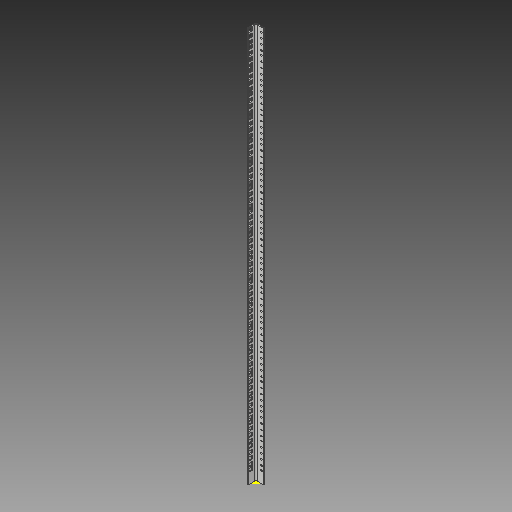
# Autodesk Inventor part: squareHoleRail20U
Saved by Autodesk Inventor 2017 (Build 210142000, 142)
## iProperties
Created: 2016-08-02
Part Number: squareHoleRail20U
Material: Generic
Document SubType Name: Sheet Metal
Designer: Zuhra Abdurashidova
Density: 1 g/cm^3
Sheet Metal Rule: Default
Appearance: Default
Author: Zuhra Abdurashidova
Autodesk Inventor part; units mm, degrees
note: some values were not read from the file. Chosen so that the rebuilt part matches the saved one: flange form of "Plate1".
ref_plane "YZ Plane" through (0, 0, 0) normal (1, 0, 0) x (0, 1, 0)
ref_plane "XZ Plane" through (0, 0, 0) normal (0, 1, 0) x (-1, 0, 0)
ref_plane "XY Plane" through (0, 0, 0) normal (0, 0, 1) x (1, 0, 0)
sketch "Sketch1" plane through (0, 0, 0) normal (0, 1, 0) x (-1, 0, 0)
  line L0 (0, 25.4) -> (0, 0)
  line L1 (0, 0) -> (-25.4, 0)
  dimension "d0" = 25.4
  dimension "d1" = 25.4
  measures "d0" distance of L0.start L0.end
  measures "d1" distance of L0.end L1.end
contour flange "Contour Flange1" sketch "Sketch1" thickness 3.048 bend radius 3.048 width 1174.75 along (0, 1, 0) mid plane no both sides no wall seen from (0, 0, 12.7) lies toward (1, 0, 0) curves L0 L1
bend "Bend1"
corner "Corner1"
sketch "Sketch2" plane through (0, 0, 25.4) normal (-1, 0, 0) x (0, 0, 1)
  line L0 (0, 1174.75) -> (0, 0) projected
  line L1 (-11.35, 1163.4) -> (-1.35, 1163.4)
  line L2 (-1.35, 1163.4) -> (-1.35, 1173.4)
  line L3 (-1.35, 1173.4) -> (-11.35, 1173.4)
  line L4 (-11.35, 1173.4) -> (-11.35, 1163.4)
  line L5 (-11.35, 1163.4) -> (-1.35, 1173.4) construction
  line L6 (-1.35, 1163.4) -> (-11.35, 1173.4) construction
  line L7 (-19.304, 1174.75) -> (0, 1174.75) projected
  line L8 (-11.35, 1147.5) -> (-1.35, 1147.5)
  line L9 (-1.35, 1147.5) -> (-1.35, 1157.5)
  line L10 (-1.35, 1157.5) -> (-11.35, 1157.5)
  line L11 (-11.35, 1157.5) -> (-11.35, 1147.5)
  line L12 (-11.35, 1147.5) -> (-1.35, 1157.5) construction
  line L13 (-1.35, 1147.5) -> (-11.35, 1157.5) construction
  line L14 (-11.35, 1131.6) -> (-1.35, 1131.6)
  line L15 (-1.35, 1131.6) -> (-1.35, 1141.6)
  line L16 (-1.35, 1141.6) -> (-11.35, 1141.6)
  line L17 (-11.35, 1141.6) -> (-11.35, 1131.6)
  line L18 (-11.35, 1131.6) -> (-1.35, 1141.6) construction
  line L19 (-1.35, 1131.6) -> (-11.35, 1141.6) construction
  line L20 (-11.35, 1118.9) -> (-1.35, 1118.9)
  line L21 (-1.35, 1118.9) -> (-1.35, 1128.9)
  line L22 (-1.35, 1128.9) -> (-11.35, 1128.9)
  line L23 (-11.35, 1128.9) -> (-11.35, 1118.9)
  line L24 (-11.35, 1118.9) -> (-1.35, 1128.9) construction
  line L25 (-1.35, 1118.9) -> (-11.35, 1128.9) construction
  point P0 (-25.4, 0)
  point P1 (-6.35, 1168.4)
  point P2 (-6.35, 1152.5)
  point P3 (-6.35, 1136.6)
  point P4 (-6.35, 1123.9)
  dimension "d13" = 6.35
  dimension "d14" = 6.35
  dimension "d15" = 10
  dimension "d16" = 10
  dimension "d17" = 15.9
  dimension "d18" = 10
  dimension "d19" = 10
  dimension "d20" = 15.9
  dimension "d21" = 10
  dimension "d22" = 10
  dimension "d23" = 12.7
  dimension "d24" = 10
  dimension "d25" = 10
  constraints: 48 end point, 8 midpoint, 8 parallel, 4 horizontal, 4 perpendicular
  measures "d13" distance from line of L0 point (-6.35, 1168.4)
  measures "d14" distance from line of L7 point (-6.35, 1168.4)
  measures "d15" distance of L3.end L1.start
  measures "d16" distance of L2.end L3.end
  measures "d17" distance of point (-6.35, 1152.5) point (-6.35, 1168.4)
  measures "d18" distance of L9.end L10.end
  measures "d19" distance of L8.end L9.end
  measures "d20" distance of point (-6.35, 1152.5) point (-6.35, 1136.6)
  measures "d21" distance of L15.end L16.end
  measures "d22" distance of L14.end L15.end
  measures "d23" distance of point (-6.35, 1123.9) point (-6.35, 1136.6)
  measures "d24" distance of L20.end L21.end
  measures "d25" distance of L21.end L22.end
extrude "Extrusion1" cut sketch "Sketch2" against normal blind 6
pattern_linear "Rectangular Pattern1" count 19 spacing 60.4 along (0, -1, 0) of "Extrusion1"
sketch "Sketch3" plane through (25.4, 0, 0) normal (0, 0, -1) x (-1, 0, 0)
  point P0 (25.4, 0)
sketch "Sketch4" plane through (25.4, 0, 0) normal (0, 0, -1) x (-1, 0, 0)
  point P0 (25.4, 0)
sketch "10-32 holes" plane through (25.4, 0, 0) normal (0, 0, -1) x (-1, 0, 0)
  circle A0 centre (6.35, 1162.05) radius 2.415
  line L0 (0, 1174.75) -> (19.304, 1174.75) projected
  line L1 (0, 0) -> (0, 1174.75) projected
  circle A1 centre (6.35, 1146.15) radius 2.415
  circle A2 centre (6.35, 1130.25) radius 2.415
  circle A3 centre (6.35, 1114.35) radius 2.415
  circle A4 centre (6.35, 1101.65) radius 2.415
  point P0 (25.4, 0)
  dimension "d31" = 4.83
  dimension "d32" = 12.7
  dimension "d33" = 6.35
  dimension "d34" = 4.83
  dimension "d35" = 15.9
  dimension "d36" = 6.35
  dimension "d37" = 4.83
  dimension "d38" = 15.9
  dimension "d39" = 4.83
  dimension "d40" = 15.9
  dimension "d41" = 4.83
  dimension "d42" = 12.7
  constraints: 5 centre point, 4 coincident
  measures "d31" diameter of A0
  measures "d32" distance from line of L0 A0.centre
  measures "d33" distance from line of L1 A0.centre
  measures "d34" diameter of A1
  measures "d35" distance of A0.centre A1.centre
  measures "d36" distance from line of L1 A1.centre
  measures "d37" diameter of A2
  measures "d38" distance of A1.centre A2.centre
  measures "d39" diameter of A3
  measures "d40" distance of A2.centre point (6.35, 1114.35)
  measures "d41" diameter of A4
  measures "d42" distance of A3.centre A4.centre
extrude "Extrusion2" cut sketch "10-32 holes" against normal blind 10
pattern_linear "Rectangular Pattern2" count 15 spacing 76.3 along (0, -1, 0) of "Extrusion2"
equation "\"d3\" = BendReliefWidth"
equation "\"d4\" = BendReliefDepth"
equation "\"d5\" = MinimumRemnant"
equation "\"d6\" = BendRadius"
equation "\"d8\" = BendRadius"
equation "\"d10\" = CornerReliefSize"
equation "\"d11\" = GapSize"
equation "\"d12\" = JacobiRadiusSize"
equation "\"BendRadius\" = Thickness"
equation "\"BendReliefWidth\" = Thickness"
equation "\"BendReliefDepth\" = 0.5 * Thickness"
equation "\"CornerReliefSize\" = 4 * Thickness"
equation "\"MinimumRemnant\" = 2 * Thickness"
equation "\"TransitionRadius\" = BendRadius"
equation "\"JacobiRadiusSize\" = Thickness"
equation "\"GapSize\" = Thickness"
equation "\"Thickness\" = 3.048"
body "Solid1"
